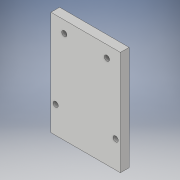
# Autodesk Inventor part: RFID Card Reader
Saved by Autodesk Inventor 2018 (Build 220112000, 112)
## iProperties
Created: 2019-09-18
Part Number: RFID Card Reader
Material: Generic
Document SubType Name: Modeling
Designer: Jacob
Density: 1 g/cm^3
Appearance: Default
Author: Jacob
Autodesk Inventor part; units mm, degrees
ref_plane "YZ Plane" through (0, 0, 0) normal (1, 0, 0) x (0, 1, 0)
ref_plane "XZ Plane" through (0, 0, 0) normal (0, 1, 0) x (-1, 0, 0)
ref_plane "XY Plane" through (0, 0, 0) normal (0, 0, 1) x (1, 0, 0)
sketch "Sketch1" plane through (0, 0, 0) normal (0, 0, 1) x (1, 0, 0)
  line L0 (-20, 30) -> (20, 30)
  line L1 (20, 30) -> (20, -30)
  line L2 (20, -30) -> (-20, -30)
  line L3 (-20, -30) -> (-20, 30)
  line L4 (-20, 30) -> (20, -30) construction
  line L5 (20, 30) -> (-20, -30) construction
  point P0 (0, 0)
  dimension "d0" = 40
  dimension "d1" = 60
  constraints: 12 end point, 2 midpoint, 2 parallel, 1 horizontal, 1 perpendicular
  measures "d0" distance of L0.start L0.end
  measures "d1" distance of L0.end L1.end
extrude "Extrusion1" add sketch "Sketch1" along normal blind 5
sketch "Sketch2" plane through (0, 0, 5) normal (0, 0, 1) x (1, 0, 0)
  line L0 (-20.0119, -14.5) -> (20, -14.5) construction
  line L1 (20, -30) -> (20, 30) projected
  line L2 (-20, -30) -> (20, -30) projected
  circle A0 centre (17.25, -14.5) radius 1.5
  circle A1 centre (-17.25, -14.5) radius 1.5
  line L3 (-20, 30) -> (-20, -30) projected
  line L4 (-20, 23.25) -> (20, 23.25) construction
  line L5 (20, 30) -> (-20, 30) projected
  circle A2 centre (12.25, 23.25) radius 1.5
  circle A3 centre (-12.25, 23.25) radius 1.5
  line L6 (0, 30) -> (0, -30) construction
  point P0 (0, 0)
  dimension "d4" = 15.5
  dimension "d5" = 3
  dimension "d6" = 3
  dimension "d9" = 6.75
  dimension "d12" = 3
  dimension "d13" = 3
  dimension "d16" = 34.5
  dimension "d17" = 17.25
  dimension "d18" = 17.25
  dimension "d19" = 24.5
  dimension "d20" = 12.25
  dimension "d21" = 12.25
  constraints: 7 point on line, 6 end point, 4 centre point, 2 horizontal, 2 midpoint
  measures "d4" distance between parallel lines of L2 L0
  measures "d5" diameter of A1
  measures "d6" diameter of A0
  measures "d9" distance between parallel lines of L5 L4
  measures "d12" diameter of A3
  measures "d13" diameter of A2
  measures "d16" distance of A0.centre A1.centre
  measures "d17" distance from line of L6 A0.centre
  measures "d18" distance from line of L6 A1.centre
  measures "d19" distance of A2.centre A3.centre
  measures "d20" distance from line of L6 A3.centre
  measures "d21" distance from line of L6 A2.centre
extrude "Extrusion2" cut sketch "Sketch2" against normal blind 25.4 contours A0 | A1 | A2 | A3
equation "\"d17\" = d18"
equation "\"d20\" = d21"
body "Solid1"
